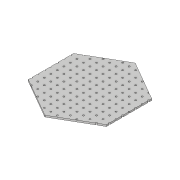
# Autodesk Inventor part: Mid_Plate
Saved by Autodesk Inventor 2017 (Build 210142000, 142)
## iProperties
Created: 2018-11-27
Part Number: Mid_Plate
Material: Generic
Document SubType Name: Modeling
Designer: jpb34
Density: 1 g/cm^3
Appearance: Default
Author: jpb34
Autodesk Inventor part; units mm, degrees
ref_plane "YZ Plane" through (0, 0, 0) normal (1, 0, 0) x (0, 1, 0)
ref_plane "XZ Plane" through (0, 0, 0) normal (0, 1, 0) x (-1, 0, 0)
ref_plane "XY Plane" through (0, 0, 0) normal (0, 0, 1) x (1, 0, 0)
sketch "Sketch1" plane through (0, 0, 0) normal (0, 1, 0) x (-1, 0, 0)
  line L0 (0, -190.5) -> (-164.9778, -95.25)
  line L1 (-164.9778, -95.25) -> (-164.9778, 95.25)
  line L2 (-164.9778, 95.25) -> (0, 190.5)
  line L3 (0, 190.5) -> (164.9778, 95.25)
  line L4 (164.9778, 95.25) -> (164.9778, -95.25)
  line L5 (164.9778, -95.25) -> (0, -190.5)
  line L6 (0, -175.8353) -> (-152.2778, -87.9177)
  line L7 (-152.2778, -87.9177) -> (-152.2778, 87.9177)
  line L8 (-152.2778, 87.9177) -> (0, 175.8353)
  line L9 (0, 175.8353) -> (152.2778, 87.9177)
  line L10 (152.2778, 87.9177) -> (152.2778, -87.9177)
  line L11 (152.2778, -87.9177) -> (0, -175.8353)
  point P0 (0, 0)
  point P1 (0, 0)
  point P2 (0, 0)
  dimension "d0" = 190.5
  dimension "d1" = 12.7
  constraints: 24 end point, 2 coincident, 26 other
  measures "d0" distance of L3.end L4.end
  measures "d1" distance between parallel lines of L4 L10
extrude "Extrusion1" add sketch "Sketch1" along normal blind 6.35 contours L6 L7 L8 L9 L10 L11
sketch "Sketch2" plane through (0, 6.35, 0) normal (0, 1, 0) x (1, 0, 0)
  circle A0 centre (0, 0) radius 3.175
  dimension "d4" = 6.35
  constraints: 1 centre point, 1 coincident
  measures "d4" diameter of A0
extrude "Extrusion2" cut sketch "Sketch2" against normal blind 12.7
pattern_linear "Rectangular Pattern1" count 20 spacing 25.4 along (1, 0, 0) count 20 spacing 25.4 along (0, 0, 1) of "Extrusion2" first direction both ways yes second direction both ways yes
sketch "Sketch3" plane through (0, 6.35, 0) normal (0, 1, 0) x (1, 0, 0)
  line L0 (152.2778, 87.9177) -> (0, 175.8353) projected
  line L1 (-152.2778, 201.4757) -> (152.2778, 201.4757)
  point P0 (0, 0)
  point P1 (-152.2778, 87.9177)
  constraints: 2 end point, 1 horizontal
body "Solid1"
